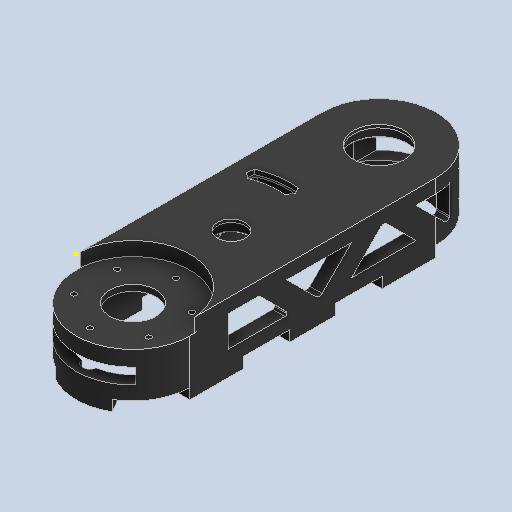
# Autodesk Inventor part: Segundo segmento - inferior - Shape generator prueba 2 - 40%
Saved by Autodesk Inventor 2026 (Build 300175050, 175E)
## iProperties
Created: 2025-07-31
Part Number: Segundo segmento - inferior - Shape generator prueba 2 - 40%
Material: Plastico PETG
Document SubType Name: Modeling
Designer: bello
Density: 1.27 g/cm^3
Appearance: Naranja
Mass: 304.449 g
Surface Area: 710.404 cm^2
Volume: 239.723 cm^3
Author: bello
Autodesk Inventor part; units mm, degrees
ref_plane "YZ Plane" through (0, 0, 0) normal (1, 0, 0) x (0, 1, 0)
sketch "Boceto1" plane through (0, 0, 0) normal (0, 1, 0) x (-1, 0, 0)
  arc A0 (37, 0) -> (-37, 0) centre (0, 0) ccw
  line L0 (37, 0) -> (37, -160)
  line L1 (-37, 0) -> (-37, -160)
  arc A1 (-37, -160) -> (37, -160) centre (0, -160) ccw
  point P0 (0, 37)
  dimension "d0" = 74
  dimension "d79" = 160
  dimension "d81" = 74
  constraints: 5 point on circle, 4 end point, 2 centre point, 2 tangent, 2 vertical, 1 coincident
  measures "d0" diameter of A0
  measures "d79" distance of L1.start L1.end
  measures "d81" diameter of A1
extrude "Extrusión1" add sketch "Boceto1" against normal blind 45
sketch "Boceto8" plane through (0, 0, 0) normal (0, 1, 0) x (1, 0, 0)
  circle A0 centre (0, 0) radius 37.1
  dimension "d48" = 74.2
  constraints: 1 centre point, 1 coincident
  measures "d48" diameter of A0
extrude "Extrusión7" cut sketch "Boceto8" against normal blind 9
sketch "Boceto9" plane through (0, -45, 0) normal (0, -1, 0) x (1, 0, 0)
  arc A0 (-29, -31.884322) -> (29, -31.884322) centre (0, 0) ccw
  arc A1 (-37, -160) -> (37, -160) centre (0, -160) ccw
  arc A2 (-29, -160) -> (29, -160) centre (0, -160) ccw
  line L0 (-37, 0) -> (-37, -160)
  line L1 (29, -160) -> (29, -31.884322)
  line L2 (-29, -160) -> (-29, -31.884322)
  dimension "d76" = 86.2
  dimension "d82" = 58
  constraints: 4 end point, 4 point on circle, 2 centre point, 2 coincident, 1 parallel, 1 vertical
  measures "d76" diameter of A0
  measures "d82" diameter of A2
extrude "Extrusión8" cut sketch "Boceto9" against normal blind 36
sketch "Boceto11" plane through (0, -45, 0) normal (0, -1, 0) x (1, 0, 0)
  arc A0 (29, 0) -> (-29, 0) centre (0, 0) ccw
  line L0 (29, 0) -> (29, -31.884322)
  arc A1 (-29, -31.884322) -> (29, -31.884322) centre (0, 0) ccw
  line L1 (-29, 0) -> (-29, -31.884322)
  arc A2 (-29, -31.884322) -> (29, -31.884322) centre (0, 0) ccw
  point P0 (-31, -182)
  dimension "d86" = 58
  constraints: 4 end point, 4 point on circle, 3 tangent, 2 centre point, 1 coincident, 1 concentric
  measures "d86" diameter of A0
extrude "Extrusión9" cut sketch "Boceto11" against normal blind 32
sketch "Boceto12" plane through (0, -13, 0) normal (0, -1, 0) x (1, 0, 0)
  circle A0 centre (0, 0) radius 28
  circle A1 centre (0, 28) radius 1.7
  circle A2 centre (-24.248711, 14) radius 1.7
  circle A3 centre (-24.248711, -14) radius 1.7
  circle A4 centre (0, -28) radius 1.7
  circle A5 centre (24.248711, -14) radius 1.7
  circle A6 centre (24.248711, 14) radius 1.7
  dimension "d60" = 56
  dimension "d61" = 3.4
  dimension "d64" = 360
  constraints: 6 centre point, 1 coincident, 1 vertical alignment, 15 other
  measures "d61" diameter of A1
extrude "Extrusión10" cut sketch "Boceto12" against normal through all contours A6 A0 | A0 A6 | A5 A0 | A0 A5 | A1 A0 | A0 A1 | A4 A0 | A0 A4 | A2 A0 | A0 A2 | A3 A0 | A0 A3
sketch "Boceto13" plane through (0, -13, 0) normal (0, -1, 0) x (1, 0, 0)
  circle A0 centre (0, 0) radius 28
  circle A1 centre (0, 28) radius 1.7
  circle A2 centre (0, 28) radius 4.7
  circle A3 centre (-24.248711, 14) radius 4.7
  circle A4 centre (-24.248711, -14) radius 4.7
  circle A5 centre (0, -28) radius 4.7
  circle A6 centre (24.248711, -14) radius 4.7
  circle A7 centre (24.248711, 14) radius 4.7
  dimension "d68" = 56
  dimension "d69" = 9.4
  dimension "d72" = 360
  constraints: 7 centre point, 2 coincident, 13 other
  measures "d68" diameter of A0
  measures "d69" diameter of A2
extrude "Extrusión11" cut sketch "Boceto13" along normal through all contours A7 A0 | A0 A7 | A2 A0 A1 | A0 A1 A2 | A1 A0 | A0 A1 | A3 A0 | A0 A3
sketch "Boceto14" plane through (0, -13, 0) normal (0, -1, 0) x (1, 0, 0)
  circle A0 centre (0, 0) radius 15
  dimension "d83" = 30
  constraints: 1 centre point, 1 coincident
  measures "d83" diameter of A0
extrude "Extrusión12" cut sketch "Boceto14" against normal through all
sketch "Boceto15" plane through (0, -45, 0) normal (0, -1, 0) x (1, 0, 0)
  arc A0 (-29, -160) -> (29, -160) centre (0, -160) ccw
  line L0 (0, -160) -> (0, 0)
  line L1 (-16.710947, -80) -> (18.438241, -80)
  line L2 (37, -160) -> (37, 0)
  line L3 (37, -35) -> (29, -35)
  line L4 (29, -35) -> (29, -65)
  line L5 (29, -65) -> (37, -65)
  line L6 (37, -65) -> (37, -35)
  line L7 (37, -95) -> (29, -95)
  line L8 (29, -95) -> (29, -125)
  line L9 (29, -125) -> (37, -125)
  line L10 (37, -125) -> (37, -95)
  circle A1 centre (0, 0) radius 15
  arc A2 (37, 0) -> (-37, 0) centre (0, 0) ccw
  line L11 (0, 0) -> (37, 0)
  line L12 (0, 0) -> (18.5, 32.04294)
  line L13 (0, -160) -> (37, -160)
  line L14 (0, -160) -> (18.5, -192.04294)
  arc A3 (-37, -160) -> (37, -160) centre (0, -160) ccw
  arc A4 (37, 0) -> (18.5, 32.04294) centre (0, 0) ccw
  arc A5 (29, 0) -> (27.117822, 10.277339) centre (0, 0) ccw
  arc A6 (29, 0) -> (14.5, 25.114737) centre (0, 0) ccw
  arc A7 (14.5, -185.114737) -> (29, -160) centre (0, -160) ccw
  arc A8 (18.5, -192.04294) -> (37, -160) centre (0, -160) ccw
  line L15 (-37, -160) -> (-37, 0)
  line L16 (-37, -35) -> (-29, -35)
  line L17 (-29, -35) -> (-29, -65)
  line L18 (-29, -65) -> (-37, -65)
  line L19 (-37, -65) -> (-37, -35)
  line L20 (-37, -95) -> (-29, -95)
  line L21 (-29, -95) -> (-29, -125)
  line L22 (-29, -125) -> (-37, -125)
  line L23 (-37, -125) -> (-37, -95)
  line L24 (0, 0) -> (-37, 0)
  line L25 (0, 0) -> (-18.5, 32.04294)
  line L26 (0, -160) -> (-37, -160)
  line L27 (0, -160) -> (-18.5, -192.04294)
  arc A9 (-18.5, 32.04294) -> (-37, 0) centre (0, 0) ccw
  arc A10 (-27.117822, 10.277339) -> (-29, 0) centre (0, 0) ccw
  arc A11 (-14.5, 25.114737) -> (-29, 0) centre (0, 0) ccw
  arc A12 (-29, -160) -> (-14.5, -185.114737) centre (0, -160) ccw
  arc A13 (-37, -160) -> (-18.5, -192.04294) centre (0, -160) ccw
  point P0 (-18.438241, -80)
  point P1 (27.117822, 10.277339)
  point P2 (-27.117822, 10.277339)
  point P3 (-18.5, 32.04294)
  point P4 (-18.5, -192.04294)
  point P5 (-14.5, -185.114737)
  dimension "d87" = 80
  dimension "d88" = 30
  dimension "d89" = 30
  dimension "d90" = 15
  dimension "d91" = 15
  dimension "d92" = 60
  dimension "d93" = 60
  constraints: 54 end point, 21 point on circle, 15 symmetric about line, 10 point on line, 9 centre point, 4 horizontal, 4 parallel, 3 concentric, 3 perpendicular, 2 tangent, 1 vertical, 5 other
  measures "d87" vertical distance of L0.end L1.end
  measures "d88" distance of L3.end L4.end
  measures "d89" distance of L7.end L8.end
  measures "d90" distance from line of L1.end L5
  measures "d91" distance from line of L1.end L7
  measures "d92" angle of L13 L14
  measures "d93" angle of L11 L12
extrude "Extrusión13" cut sketch "Boceto15" against normal blind 7 contours A0 L27 A3 L26 | A0 L13 A3 L14 | L15 L20 L21 L22 | L9 L8 L7 L2 | L15 L16 L17 L18 | L24 A2 L25 A11 A10 | A5 A6 L12 A2 L11 | L5 L4 L3 L2
sketch "Boceto16" plane through (0, -38, 0) normal (0, -1, 0) x (1, 0, 0)
  circle A0 centre (33, -50) radius 2.05
  circle A1 centre (33, -110) radius 2.05
  circle A2 centre (0, 0) radius 33
  circle A3 centre (21.211991, 25.279467) radius 2.05
  arc A4 (-29, -160) -> (29, -160) centre (0, -160) ccw
  circle A5 centre (0, -160) radius 33
  circle A6 centre (28.578838, -176.5) radius 2.05
  line L0 (37, -35) -> (37, -65)
  line L1 (37, -65) -> (29, -65)
  line L2 (29, -95) -> (37, -95)
  line L3 (37, -95) -> (37, -125)
  line L4 (28.578838, -176.5) -> (0, -160)
  line L5 (0, -160) -> (18.249621, -160)
  line L6 (0, 0) -> (21.211991, 25.279467)
  line L7 (0, 0) -> (19.878648, 0)
  line L8 (0, 0) -> (0, -160)
  circle A7 centre (-33, -50) radius 2.05
  circle A8 centre (-33, -110) radius 2.05
  circle A9 centre (-21.211991, 25.279467) radius 2.05
  circle A10 centre (-28.578838, -176.5) radius 2.05
  line L9 (-28.578838, -176.5) -> (0, -160)
  line L10 (0, 0) -> (-21.211991, 25.279467)
  dimension "d96" = 66
  dimension "d97" = 66
  dimension "d98" = 4.1
  dimension "d99" = 4
  dimension "d100" = 15
  dimension "d101" = 15
  dimension "d102" = 4
  dimension "d103" = 50
  dimension "d104" = 30
  constraints: 14 end point, 8 centre point, 4 symmetric about line, 3 equal radius, 2 coincident, 2 horizontal, 1 vertical, 10 other
  measures "d98" diameter of A0
  measures "d99" distance from line of L0 A0.centre
  measures "d100" distance from line of L1 A0.centre
  measures "d101" distance from line of L2 A1.centre
  measures "d102" distance from line of L3 A1.centre
  measures "d103" angle of L7 L6
  measures "d104" angle of L4 L5
extrude "Extrusión14" cut sketch "Boceto16" against normal blind 5.8 contours A0 | A1 | A3 L6 A2 | A2 A3 | L6 A3 A2 | A9 A2 | A2 L10 A9 | A2 A9 L10 | L9 A5 A10 | A10 A5 L9 | L4 A5 A6 | A6 A5 L4 | A5 A10 | A6 A5 | A7 | A8
sketch "Boceto17" plane through (0, -9, 0) normal (0, -1, 0) x (1, 0, 0)
  arc A0 (14.5, -185.114737) -> (29, -160) centre (0, -160) ccw
  circle A1 centre (0, -160) radius 16.5
  circle A2 centre (0, -64) radius 9
  point P0 (0, 0)
  dimension "d107" = 96
  dimension "d108" = 33
  dimension "d109" = 18
  constraints: 2 centre point, 1 coincident
  measures "d107" distance of A2.centre A1.centre
  measures "d108" diameter of A1
  measures "d109" diameter of A2
extrude "Extrusión15" cut sketch "Boceto17" against normal through all
sketch "Boceto18" plane through (0, -9, 0) normal (0, -1, 0) x (1, 0, 0)
  circle A0 centre (0, -64) radius 9 projected
  circle A1 centre (0, -64) radius 11
  circle A2 centre (0, -160) radius 16.5 projected
  circle A3 centre (0, -160) radius 16.5
  circle A4 centre (0, -160) radius 18.5
  point P0 (0, 0)
  dimension "d112" = 22
  dimension "d206" = 37
  constraints: 3 centre point, 3 coincident
  measures "d112" diameter of A1
  measures "d206" diameter of A4
extrude "Extrusión16" cut sketch "Boceto18" against normal blind 7
sketch "Boceto19" plane through (0, -9, 0) normal (0, -1, 0) x (1, 0, 0)
  circle A0 centre (0, -160) radius 16.5 projected
  circle A1 centre (0, -160) radius 22.5
  point P0 (0, 0)
  dimension "d115" = 45
  constraints: 1 centre point, 1 coincident
  measures "d115" diameter of A1
split_face "Dividir1"
sketch "Boceto20" plane through (-37, 0, -160) normal (-1, 0, 0) x (0, 0, 1)
  point P0 (160, 0)
ref_plane "Plano de trabajo1" through (37, 0, 0) normal (0, 0, -1) x (0, -1, 0)
sketch "Boceto21" plane through (37, 0, 0) normal (0, 0, -1) x (0, -1, 0)
  line L0 (44.659186, 37) -> (-6.659186, 37)
  line L1 (9, 48) -> (9, 26)
  line L2 (29, 10) -> (29, 37)
  line L3 (29, 37) -> (29, 64)
  line L4 (29, 64) -> (19, 64)
  line L5 (19, 64) -> (19, 37)
  line L6 (19, 10) -> (29, 10)
  line L7 (19, 37) -> (19, 10)
  line L8 (45, 18.5) -> (45, 55.5)
  point P0 (0, 37)
  dimension "d118" = 27
  dimension "d119" = 10
  dimension "d120" = 16
  constraints: 14 end point, 5 perpendicular, 2 equal length, 2 point on line, 1 horizontal, 1 midpoint, 1 vertical
  measures "d118" distance of L2.end L3.end
  measures "d119" distance of L3.end L4.end
  measures "d120" distance between parallel lines of L8 L3
extrude "Extrusión17" cut sketch "Boceto21" along normal through all both and the other way through all
sketch "Boceto22" plane through (-37, 0, -160) normal (-1, 0, 0) x (0, 0, 1)
  line L0 (114.9, -9) -> (97.22233, -26.67767)
  line L1 (114.9, -9) -> (134.9, -9)
  line L2 (134.9, -9) -> (134.9, -29)
  line L3 (77.808117, -28.091883) -> (96.9, -9)
  line L4 (73.991883, -28.091883) -> (54.9, -9)
  line L5 (96.9, -9) -> (54.9, -9)
  line L6 (0, 0) -> (157.277868, 0)
  arc A0 (73.991883, -28.091883) -> (77.808117, -28.091883) centre (75.9, -26.183766) ccw
  line L7 (54.9, -9) -> (54.9, -31.916229)
  line L8 (54.9, -28.882251) -> (12.9, -28.882251)
  line L9 (12.9, -28.882251) -> (31.991883, -9.790368)
  line L10 (54.9, -28.882251) -> (35.808117, -9.790368)
  arc A1 (35.808117, -9.790368) -> (31.991883, -9.790368) centre (33.9, -11.698485) ccw
  line L11 (12.9, -28.882251) -> (12.9, -16.233544)
  line L12 (12.9, -16.233544) -> (12.9, -9)
  line L13 (128.115678, -9) -> (0, -9)
  line L14 (12.9, -9) -> (-29.1, -9)
  line L15 (12.9, -9) -> (-6.191883, -28.091883)
  arc A2 (-10.008117, -28.091883) -> (-6.191883, -28.091883) centre (-8.1, -26.183766) ccw
  line L16 (-10.583005, -19) -> (-10.583005, -29)
  line L17 (-10.583005, -27.516995) -> (-10.583005, -9)
  line L18 (-10.583005, -27.516995) -> (-10.008117, -28.091883)
  line L19 (96.9, -9) -> (96.9, -29)
  line L20 (134.9, -29) -> (98.184271, -29)
  arc A3 (97.22233, -26.67767) -> (98.184271, -29) centre (98.184271, -27.63961) ccw
  point P0 (160, 0)
  point P1 (75.9, -28.882251)
  point P2 (-19.1, -9)
  point P3 (96.9, -27.190937)
  point P4 (96.9, -28.088283)
  dimension "d131" = 135
  dimension "d132" = 20
  dimension "d134" = 45
  dimension "d135" = 45
  dimension "d140" = 18
  dimension "d141" = 42
  dimension "d156" = 27
  dimension "d157" = 19.88225
  dimension "d165" = 27
  dimension "d166" = 45
  dimension "d167" = 45
  dimension "d168" = 42
  dimension "d169" = 27
  dimension "d170" = 45
  dimension "d172" = 42
  dimension "d179" = 20
  dimension "d180" = 25
  constraints: 36 end point, 9 point on circle, 6 point on line, 5 tangent, 4 centre point, 4 perpendicular, 3 horizontal, 3 vertical, 1 other
  measures "d131" angle of L1 L0
  measures "d132" distance of L1.end L2.end
  measures "d134" angle of L5 L4
  measures "d135" angle of L5 L3
  measures "d140" distance of L0.start L3.end
  measures "d141" distance of L3.end L4.end
  measures "d156" distance of L3.start L3.end
  measures "d157" distance from line of L5 point (75.9, -28.882)
  measures "d165" distance of L8.start L10.end
  measures "d166" angle of L8 L10
  measures "d167" angle of L8 L9
  measures "d168" distance of L8.start L8.end
  measures "d169" distance of L12.end L15.end
  measures "d170" angle of L14 L15
  measures "d172" distance of L12.end L14.end
  measures "d179" distance of L0.start L1.end
  measures "d180" distance of L0.start L0.end
extrude "Extrusión18" cut sketch "Boceto22" against normal blind 8 contours L1 L2 L20 A3 L19 L0 | L15 A2 L18 L16 L17 L14 L13 | L3 A0 L4 L5 | L8 L9 A1 L10
ref_plane "Plano de trabajo2" through (0, -13, -31.884322) normal (-1, 0, 0) x (0, 0, 1)
mirror "Simetría1" about plane through (0, -13, -31.884322) normal (-1, 0, 0) of "Extrusión18"
sketch "Boceto23" plane through (-29, 0, -160) normal (-1, 0, 0) x (0, 0, 1)
  line L0 (-10.583005, -9) -> (0, -9)
  line L1 (0, -9) -> (-10.583005, -9)
  line L2 (-10.583005, -27.516995) -> (-10.583005, -9)
  line L3 (-10.583005, -9) -> (-10.583005, -27.516995)
  line L4 (0, -21.9) -> (0, -9)
  line L5 (0, -9) -> (0, -21.9)
  arc A0 (-10.008117, -28.091883) -> (-6.191883, -28.091883) centre (-8.1, -26.183766) ccw
  line L6 (0, -21.9) -> (-6.191883, -28.091883)
  arc A1 (-10.008117, -28.091883) -> (-6.191883, -28.091883) centre (-8.1, -26.183766) ccw
  line L7 (-10.583005, -27.516995) -> (-10.008117, -28.091883)
  line L8 (-10.583005, -27.516995) -> (-10.008117, -28.091883)
  point P0 (160, 0)
  constraints: 10 end point, 3 collinear, 3 tangent, 2 point on circle, 1 centre point, 1 perpendicular
extrude "Extrusión19" cut sketch "Boceto23" against normal blind 8
mirror "Simetría2" about plane through (0, -13, -31.884322) normal (-1, 0, 0) of "Extrusión19"
sketch "Boceto25" plane through (37, -45, -160) normal (0, 0, -1) x (-1, 0, 0)
  line L0 (64, 26) -> (10, 26)
  line L1 (10, 26) -> (10, 33)
  line L2 (10, 33) -> (64, 33)
  line L3 (64, 33) -> (64, 26)
  line L4 (10, 16) -> (10, 26) projected
  point P0 (37, 45)
  dimension "d175" = 0
  dimension "d176" = 7
  constraints: 8 end point, 2 parallel, 1 horizontal, 1 perpendicular
  measures "d175" distance between parallel lines of L4 L1
  measures "d176" distance of L2.end L0.start
extrude "Extrusión20" cut sketch "Boceto25" along normal through all
sketch "Boceto29" plane through (-35.454196, -9, -170.583005) normal (0, -1, 0) x (1, 0, 0)
  circle A0 centre (35.454196, 106.583005) radius 11
  circle A1 centre (35.454196, 106.583005) radius 8
  circle A2 centre (35.454196, 10.583005) radius 16.5
  circle A3 centre (35.454196, 10.583005) radius 26
  line L0 (27.596079, 108.083005) -> (9.915316, 15.458005)
  line L1 (43.312313, 108.083005) -> (60.993075, 15.458005)
  line L2 (27.596079, 108.083005) -> (11.611183, 66.017781)
  line L3 (27.596079, 108.083005) -> (30.886375, 63.203456)
  circle A4 centre (27.596079, 108.083005) radius 43.4
  circle A5 centre (30.769387, 64.799173) radius 2.6
  circle A6 centre (12.179535, 67.513433) radius 2.6
  circle A7 centre (27.596079, 108.083005) radius 40.8
  circle A8 centre (27.596079, 108.083005) radius 46
  point P0 (35.454196, 170.583005)
  point P1 (30.579281, 67.392214)
  point P2 (13.103107, 69.943869)
  point P3 (11.255963, 65.082998)
  point P4 (30.959493, 62.206133)
  dimension "d191" = 16
  dimension "d192" = 52
  dimension "d195" = 10
  dimension "d196" = 15
  dimension "d214" = 5.2
  dimension "d215" = 5.2
  constraints: 8 end point, 7 centre point, 6 point on circle, 5 coincident, 4 tangent, 2 point on line
  measures "d191" diameter of A1
  measures "d192" diameter of A3
  measures "d195" angle of L0 L2
  measures "d196" angle of L3 L0
  measures "d214" diameter of A5
  measures "d215" diameter of A6
extrude "Extrusión23" cut sketch "Boceto29" against normal through all contours A6 A4 L2 | A7 L0 A4 A6 | L2 A4 A6 | A7 A5 A4 L0 | A4 A6 | A5 A4 L3 | L3 A4 A5 | A4 A5 A8 L0 | L0 A8 A6 A4 | A4 A5
sketch "Boceto30" plane through (0, 0, 0) normal (0, 1, 0) x (1, 0, 0)
  line L0 (-4.911927, 109.81028) -> (-2.089726, 109.603373)
  line L1 (-2.089726, 109.603373) -> (-0.079447, 105.446195)
  line L2 (-0.079447, 105.446195) -> (-2.674531, 101.626654)
  line L3 (-2.674531, 101.626654) -> (-4.977211, 101.795472)
  line L4 (-24.01257, 98.510096) -> (-27.592238, 101.428881)
  line L5 (-27.592238, 101.428881) -> (-26.854329, 105.988358)
  line L6 (-26.854329, 105.988358) -> (-24.29605, 106.96051)
  line L7 (-22.107628, 99.233979) -> (-24.01257, 98.510096)
  arc A0 (-4.977211, 101.795472) -> (-22.107628, 99.233979) centre (-7.858117, 62.5) ccw
  arc A1 (-2.062099, 109.546241) -> (-26.86465, 105.924582) centre (-7.858117, 62.5) ccw
  point P0 (0, 0)
  point P1 (-23.274661, 103.069572)
  point P2 (-4.684809, 105.783832)
  point P3 (-4.684809, 105.783832)
  point P4 (-23.274661, 103.069572)
  dimension "d203" = 8
  constraints: 16 end point, 6 point on circle, 3 coincident, 2 centre point, 2 point on line, 12 other
  measures "d203" distance between parallel lines of L6 L7
sketch "Boceto30 outline for Extrusión24" plane through (0, 0, 0) normal (0, 1, 0) x (1, 0, 0)
  line L0 (-27.592238, 101.428881) -> (-24.01257, 98.510096)
  line L1 (-26.86465, 105.924582) -> (-27.592238, 101.428881)
  arc A0 (-2.062099, 109.546241) -> (-26.86465, 105.924582) centre (-7.858117, 62.5) ccw
  line L2 (-0.079447, 105.446195) -> (-2.062099, 109.546241)
  line L3 (-2.674531, 101.626654) -> (-0.079447, 105.446195)
  line L4 (-4.977211, 101.795472) -> (-2.674531, 101.626654)
  arc A1 (-22.107628, 99.233979) -> (-4.977211, 101.795472) centre (-7.858117, 62.5) cw
  line L5 (-24.01257, 98.510096) -> (-22.107628, 99.233979)
extrude "Extrusión24" cut sketch "Boceto30 outline for Extrusión24" against normal blind 3
chamfer "Chaflán1" distance 0.7 angle 45 2 edges at (-11, -9, -64) (-18.5, -9, -160)
equation "\"d9\" = Altura"
equation "\"Altura\" = 45"
